Autodesk Fusion 360 part; units mm, degrees
note: some values were not read from the file. Set by a fixed rule: which face or edge a step refers to.
(part 3 of 5)
sketch "Sketch2 (10)" plane through (0, -26.65, 0) normal (0, -1, 0) x (1, 0, 0) in component "Front_R_Mounting_Plate"
  circle A0 centre (3, -97) radius 1.0625
  circle A1 centre (3, -71) radius 1.0625
  circle A2 centre (22, -71) radius 1.0625
  circle A3 centre (3, -29) radius 1.0625
  circle A4 centre (3, -3) radius 1.0625
  circle A5 centre (22, -29) radius 1.0625
  circle A6 centre (90, -16) radius 1.0625
  circle A7 centre (114, -16) radius 1.0625
  circle A8 centre (90, -30.28) radius 1.0625
  circle A9 centre (114, -30.28) radius 1.0625
  circle A10 centre (114, -69.72) radius 1.0625
  circle A11 centre (90, -84) radius 1.0625
  circle A12 centre (90, -69.72) radius 1.0625
  circle A13 centre (114, -84) radius 1.0625
  line L0 (92.5, -27.97) -> (92.5, -18.97)
  line L1 (92.5, -18.97) -> (112.5, -18.97)
  line L2 (112.5, -18.97) -> (112.5, -27.97)
  line L3 (112.5, -27.97) -> (92.5, -27.97)
  circle A14 centre (11.5, -70.07) radius 1
  circle A15 centre (11.5, -4.1) radius 1
  circle A16 centre (11.5, -29.93) radius 1
  line L4 (92.5, -81.36) -> (92.5, -72.36)
  line L5 (92.5, -72.36) -> (112.5, -72.36)
  line L6 (112.5, -72.36) -> (112.5, -81.36)
  line L7 (112.5, -81.36) -> (92.5, -81.36)
  circle A17 centre (89.585, -23.47) radius 1
  circle A18 centre (115.415, -76.86) radius 1
  line L8 (16, -72.97) -> (16, -93)
  line L9 (16, -93) -> (7, -93)
  line L10 (7, -93) -> (7, -72.97)
  line L11 (7, -72.97) -> (16, -72.97)
  line L12 (16, -7) -> (16, -27.03)
  line L13 (16, -27.03) -> (7, -27.03)
  line L14 (7, -27.03) -> (7, -7)
  line L15 (7, -7) -> (16, -7)
  circle A19 centre (11.5, -95.9) radius 1
  circle A20 centre (89.585, -76.86) radius 1
  circle A21 centre (115.415, -23.47) radius 1
  line L16 (127.5, -73.5) -> (124.5, -73.5)
  line L17 (124.5, -73.5) -> (124.5, -68.5)
  line L18 (124.5, -68.5) -> (127.5, -68.5)
  line L19 (127.5, -68.5) -> (127.5, -73.5)
  line L20 (183.5, -73.5) -> (180.5, -73.5)
  line L21 (180.5, -73.5) -> (180.5, -68.5)
  line L22 (180.5, -68.5) -> (183.5, -68.5)
  line L23 (183.5, -68.5) -> (183.5, -73.5)
  line L24 (127.5, -31.5) -> (124.5, -31.5)
  line L25 (124.5, -31.5) -> (124.5, -26.5)
  line L26 (124.5, -26.5) -> (127.5, -26.5)
  line L27 (127.5, -26.5) -> (127.5, -31.5)
  line L28 (183.5, -31.5) -> (180.5, -31.5)
  line L29 (180.5, -31.5) -> (180.5, -26.5)
  line L30 (180.5, -26.5) -> (183.5, -26.5)
  line L31 (183.5, -26.5) -> (183.5, -31.5)
  arc A22 (157, -3) -> (154, 0) centre (154, -3) ccw
  line L32 (154, 0) -> (3, 0)
  arc A23 (3, 0) -> (0, -3) centre (3, -3) ccw
  line L33 (0, -3) -> (0, -97)
  arc A24 (0, -97) -> (3, -100) centre (3, -97) ccw
  line L34 (3, -100) -> (154, -100)
  arc A25 (154, -100) -> (157, -97) centre (154, -97) ccw
  line L35 (157, -97) -> (157, -94)
  arc A26 (160, -91) -> (157, -94) centre (160, -94) ccw
  line L36 (160, -91) -> (181.27, -91)
  arc A27 (181.27, -91) -> (184.27, -88) centre (181.27, -88) ccw
  line L37 (184.27, -88) -> (184.27, -12)
  arc A28 (184.27, -12) -> (181.27, -9) centre (181.27, -12) ccw
  line L38 (181.27, -9) -> (160, -9)
  arc A29 (157, -6) -> (160, -9) centre (160, -6) ccw
  line L39 (157, -6) -> (157, -3)
  line L40 (36.83, -3.81) -> (36.83, -13.97)
  line L41 (36.83, -13.97) -> (19.05, -13.97)
  line L42 (19.05, -13.97) -> (19.05, -3.81)
  line L43 (19.05, -3.81) -> (36.83, -3.81)
  line L44 (36.83, -96.52) -> (19.05, -96.52)
  line L45 (19.05, -96.52) -> (19.05, -86.36)
  line L46 (19.05, -86.36) -> (36.83, -86.36)
  line L47 (36.83, -86.36) -> (36.83, -96.52)
  line L48 (114.3, -3.81) -> (130.81, -3.81)
  line L49 (130.81, -3.81) -> (130.81, -13.97)
  line L50 (130.81, -13.97) -> (114.3, -13.97)
  line L51 (114.3, -13.97) -> (114.3, -3.81)
  line L52 (114.3, -96.52) -> (114.3, -86.36)
  line L53 (114.3, -86.36) -> (130.81, -86.36)
  line L54 (130.81, -86.36) -> (130.81, -96.52)
  line L55 (130.81, -96.52) -> (114.3, -96.52)
  line L56 (25, -13.97) -> (25, -31.97)
  line L57 (25, -31.97) -> (0, -31.97)
  line L58 (0, -31.97) -> (0, -3)
  line L59 (19.05, -3.81) -> (19.05, 0)
  line L60 (19.05, 0) -> (3, 0)
  arc A30 (3, 0) -> (0, -3) centre (3, -3) ccw
  line L61 (19.05, -3.81) -> (19.05, -13.97)
  line L62 (19.05, -13.97) -> (25, -13.97)
  line L63 (7, -27.03) -> (7, -15.03) construction
  line L64 (7, -15.03) -> (16, -15.03)
  dimension "d323" = 25
  dimension "d324" = 18
  dimension "d325" = 3
  dimension "d326" = 12
  constraint coincident L41 L56.start
  constraint perpendicular L41 L56
  constraint coincident L33 L57.end
  constraint perpendicular L33 L57
  constraint coincident A23.end L33.start
  constraint coincident L42.end L43.start
  constraint coincident L32 L59.end
  constraint perpendicular L32 L59
  constraint coincident L32.end A23.start
  constraint coincident L41.end L42.start
  constraint coincident L13.end L14.start
  constraint perpendicular L13 L63
  constraint coincident L12 L64.end
  constraint perpendicular L12 L64
  measures "d323" distance of L56.end L57.end
  measures "d324" distance of L56.start L56.end
  measures "d325" radius of A30
  measures "d326" distance of L13.end L63.end
extrude "Extrude1''''''''''" add sketch "Sketch2 (10)" along normal blind 5.45 separate body contours A3 | A4 | A5 | L12 L14 L15 L64 | L32 A23 L33 L41 L42 L56 L57 L58 L59 L60 A30 L61 L62 makes body 15 in component "Front_R_Mounting_Plate"
sketch "Sketch3 (6)" plane through (0, -32.1, 0) normal (0, -1, 0) x (1, 0, 0) in component "Front_R_Mounting_Plate"
  line L0 (7, -27.03) -> (7, -15.03)
  line L1 (7, -15.03) -> (16, -15.03)
  line L2 (16, -15.03) -> (16, -27.03)
  line L3 (16, -27.03) -> (7, -27.03)
  line L4 (19.05, -13.97) -> (19.05, 0)
  line L5 (19.05, 0) -> (3, 0)
  arc A0 (3, 0) -> (0, -3) centre (3, -3) ccw
  line L6 (0, -3) -> (0, -31.97)
  line L7 (0, -31.97) -> (25, -31.97)
  line L8 (25, -31.97) -> (25, -13.97)
  line L9 (25, -13.97) -> (19.05, -13.97)
  line L10 (11.5, -27.03) -> (11.5, -23.23) construction
  circle A1 centre (11.5, -23.23) radius 8.2
  circle A2 centre (11.5, -23.23) radius 10.2
  circle A3 centre (11.5, -4.1) radius 1
  circle A4 centre (11.5, -29.93) radius 1
  dimension "d329" = 3.8
  dimension "d330" = 16.4
  dimension "d331" = 2
  constraint midpoint L3 L10.start
  constraint perpendicular L3 L10
  constraint coincident L10.end A1.centre
  measures "d329" distance of L10.start L10.end
  measures "d330" diameter of A1
extrude "Extrude2''''''''" cut sketch "Sketch3 (6)" against normal blind 2 contours L7 A2 picked at (9.2691, -14.4428) bodies 15 in component "Front_R_Mounting_Plate"
sketch "Sketch4 (7)" plane through (0, -26.65, 0) normal (0, -1, 0) x (1, 0, 0) in component "Front_R_Mounting_Plate"
  circle A0 centre (3, -97) radius 1.0625
  circle A1 centre (3, -71) radius 1.0625
  circle A2 centre (22, -71) radius 1.0625
  circle A3 centre (3, -29) radius 1.0625
  circle A4 centre (3, -3) radius 1.0625
  circle A5 centre (22, -29) radius 1.0625
  circle A6 centre (90, -16) radius 1.0625
  circle A7 centre (114, -16) radius 1.0625
  circle A8 centre (90, -30.28) radius 1.0625
  circle A9 centre (114, -30.28) radius 1.0625
  circle A10 centre (114, -69.72) radius 1.0625
  circle A11 centre (90, -84) radius 1.0625
  circle A12 centre (90, -69.72) radius 1.0625
  circle A13 centre (114, -84) radius 1.0625
  line L0 (92.5, -27.97) -> (92.5, -18.97)
  line L1 (92.5, -18.97) -> (112.5, -18.97)
  line L2 (112.5, -18.97) -> (112.5, -27.97)
  line L3 (112.5, -27.97) -> (92.5, -27.97)
  circle A14 centre (11.5, -70.07) radius 1
  circle A15 centre (11.5, -4.1) radius 1
  circle A16 centre (11.5, -29.93) radius 1
  line L4 (92.5, -81.36) -> (92.5, -72.36)
  line L5 (92.5, -72.36) -> (112.5, -72.36)
  line L6 (112.5, -72.36) -> (112.5, -81.36)
  line L7 (112.5, -81.36) -> (92.5, -81.36)
  circle A17 centre (89.585, -23.47) radius 1
  circle A18 centre (115.415, -76.86) radius 1
  line L8 (16, -72.97) -> (16, -93)
  line L9 (16, -93) -> (7, -93)
  line L10 (7, -93) -> (7, -72.97)
  line L11 (7, -72.97) -> (16, -72.97)
  line L12 (16, -7) -> (16, -27.03)
  line L13 (16, -27.03) -> (7, -27.03)
  line L14 (7, -27.03) -> (7, -7)
  line L15 (7, -7) -> (16, -7)
  circle A19 centre (11.5, -95.9) radius 1
  circle A20 centre (89.585, -76.86) radius 1
  circle A21 centre (115.415, -23.47) radius 1
  line L16 (127.5, -73.5) -> (124.5, -73.5)
  line L17 (124.5, -73.5) -> (124.5, -68.5)
  line L18 (124.5, -68.5) -> (127.5, -68.5)
  line L19 (127.5, -68.5) -> (127.5, -73.5)
  line L20 (183.5, -73.5) -> (180.5, -73.5)
  line L21 (180.5, -73.5) -> (180.5, -68.5)
  line L22 (180.5, -68.5) -> (183.5, -68.5)
  line L23 (183.5, -68.5) -> (183.5, -73.5)
  line L24 (127.5, -31.5) -> (124.5, -31.5)
  line L25 (124.5, -31.5) -> (124.5, -26.5)
  line L26 (124.5, -26.5) -> (127.5, -26.5)
  line L27 (127.5, -26.5) -> (127.5, -31.5)
  line L28 (183.5, -31.5) -> (180.5, -31.5)
  line L29 (180.5, -31.5) -> (180.5, -26.5)
  line L30 (180.5, -26.5) -> (183.5, -26.5)
  line L31 (183.5, -26.5) -> (183.5, -31.5)
  arc A22 (157, -3) -> (154, 0) centre (154, -3) ccw
  line L32 (154, 0) -> (3, 0)
  arc A23 (3, 0) -> (0, -3) centre (3, -3) ccw
  line L33 (0, -3) -> (0, -97)
  arc A24 (0, -97) -> (3, -100) centre (3, -97) ccw
  line L34 (3, -100) -> (154, -100)
  arc A25 (154, -100) -> (157, -97) centre (154, -97) ccw
  line L35 (157, -97) -> (157, -94)
  arc A26 (160, -91) -> (157, -94) centre (160, -94) ccw
  line L36 (160, -91) -> (181.27, -91)
  arc A27 (181.27, -91) -> (184.27, -88) centre (181.27, -88) ccw
  line L37 (184.27, -88) -> (184.27, -12)
  arc A28 (184.27, -12) -> (181.27, -9) centre (181.27, -12) ccw
  line L38 (181.27, -9) -> (160, -9)
  arc A29 (157, -6) -> (160, -9) centre (160, -6) ccw
  line L39 (157, -6) -> (157, -3)
  line L40 (36.83, -3.81) -> (36.83, -13.97)
  line L41 (36.83, -13.97) -> (19.05, -13.97)
  line L42 (19.05, -13.97) -> (19.05, -3.81)
  line L43 (19.05, -3.81) -> (36.83, -3.81)
  line L44 (36.83, -96.52) -> (19.05, -96.52)
  line L45 (19.05, -96.52) -> (19.05, -86.36)
  line L46 (19.05, -86.36) -> (36.83, -86.36)
  line L47 (36.83, -86.36) -> (36.83, -96.52)
  line L48 (114.3, -3.81) -> (130.81, -3.81)
  line L49 (130.81, -3.81) -> (130.81, -13.97)
  line L50 (130.81, -13.97) -> (114.3, -13.97)
  line L51 (114.3, -13.97) -> (114.3, -3.81)
  line L52 (114.3, -96.52) -> (114.3, -86.36)
  line L53 (114.3, -86.36) -> (130.81, -86.36)
  line L54 (130.81, -86.36) -> (130.81, -96.52)
  line L55 (130.81, -96.52) -> (114.3, -96.52)
  circle A30 centre (3, -29) radius 1.0625
  circle A31 centre (22, -29) radius 1.0625
  circle A32 centre (3, -3) radius 1.0625
  circle A33 centre (3, -3) radius 1.0625
  circle A34 centre (3, -3) radius 1.0625
  circle A35 centre (22, -29) radius 1.0625
  circle A36 centre (3, -29) radius 1.0625
  circle A37 centre (3, -3) radius 1.0625
  circle A38 centre (3, -3) radius 1.0625
  circle A39 centre (3, -3) radius 0.95
  circle A40 centre (3, -29) radius 0.95
  circle A41 centre (22, -29) radius 0.95
  dimension "d334" = 1.9
  dimension "d335" = 1.9
  dimension "d336" = 1.9
  constraint concentric A36 A40
  constraint concentric A35 A41
  measures "d334" diameter of A39
  measures "d335" diameter of A40
  measures "d336" diameter of A41
extrude "Extrude3''''''" add sketch "Sketch4 (7)" against normal blind 1 contours A39 | A40 | A41 bodies 15 in component "Front_R_Mounting_Plate"
sketch "Sketch6 (4)" plane through (0, -26.65, 0) normal (0, 1, 0) x (-1, 0, 0) in component "Front_R_Mounting_Plate"
  circle A0 centre (-22, -29) radius 0.95
  circle A1 centre (-3, -3) radius 0.95
  circle A2 centre (-3, -29) radius 0.95
  line L0 (-7, -15.03) -> (-7, -27.03)
  line L1 (-7, -27.03) -> (-16, -27.03)
  line L2 (-16, -27.03) -> (-16, -15.03)
  line L3 (-16, -15.03) -> (-7, -15.03)
  line L4 (-19.05, 0) -> (-19.05, -13.97)
  line L5 (-19.05, -13.97) -> (-25, -13.97)
  line L6 (-25, -13.97) -> (-25, -31.97)
  line L7 (-25, -31.97) -> (0, -31.97)
  line L8 (0, -31.97) -> (0, -3)
  arc A3 (0, -3) -> (-3, 0) centre (-3, -3) ccw
  line L9 (-3, 0) -> (-19.05, 0)
  line L10 (-17.55, 0) -> (-5.45, 0)
  line L11 (-5.45, 0) -> (-5.45, -31.97)
  line L12 (-17.55, -31.97) -> (-17.55, 0)
  line L13 (-17.55, 0) -> (-8.3527, -31.97) construction
  line L14 (-5.45, 0) -> (-14.6473, -31.97) construction
  line L15 (-5.45, -31.97) -> (-17.55, -31.97)
  circle A4 centre (-11.5, -4.1) radius 1
  circle A5 centre (-11.5, -29.93) radius 1
  point P0 (-11.5, -21.03)
  dimension "d340" = 7.45
  dimension "d341" = 5.45
  constraint horizontal L10
  constraint perpendicular L10 L11
  constraint parallel L11 L12
  constraint coincident L13 P0
  constraint coincident L14 P0
  constraint coincident L7 L14.end
  constraint coincident L7 L13.end
  constraint coincident L7 L11.end
  constraint coincident L7 L12.start
  measures "d340" distance of L6 L12
  measures "d341" distance of L8 L11
extrude "Extrude4''''''" cut sketch "Sketch6 (4)" against normal blind 1.5 contours L7 L9 L10 L11 L12 L15 | A4 | A5 bodies 15 in component "Front_R_Mounting_Plate"
extrude "Extrude18''" add 4 faces at (92.6744, -34.28, -80.7632) (100.2032, -34.28, -80.4856) (99.9256, -34.28, -72.9568) (92.3968, -34.28, -73.2344) along direction (0, 1, 0) blind 1.8 on bodies 12 bodies 12 in component "Back_Wheel_L"
extrude "Extrude19''" add 8 faces at (91.0152, -35.28, -77.0342) (94.3333, -35.28, -74.9002) (96.4742, -35.28, -71.5752) (98.2598, -35.28, -74.8933) (101.59, -35.28, -76.86) (98.2598, -35.28, -78.8267) (96.4742, -35.28, -82.1448) (94.3333, -35.28, -78.8198) along direction (0, 1, 0) blind 1.8 on bodies 12 bodies 12 in component "Back_Wheel_L"
extrude "Extrude20'" add 4 faces at (92.6744, -34.28, -80.7632) (100.2032, -34.28, -80.4856) (99.9256, -34.28, -72.9568) (92.3968, -34.28, -73.2344) along direction (0, 1, 0) blind 1.8 on bodies 13 bodies 13 in component "Back_Wheel_R"
extrude "Extrude21" add 8 faces at (91.0152, -35.28, -77.0342) (94.3333, -35.28, -74.9002) (96.4742, -35.28, -71.5752) (98.2598, -35.28, -74.8933) (101.59, -35.28, -76.86) (98.2598, -35.28, -78.8267) (96.4742, -35.28, -82.1448) (94.3333, -35.28, -78.8198) along direction (0, 1, 0) blind 1.8 on bodies 13 bodies 13 in component "Back_Wheel_R"
sketch "Sketch50" plane through (0, -33.48, 0) normal (0, 1, 0) x (-1, 0, 0)
  circle A0 centre (-96.3, -76.86) radius 2.25
  arc A1 (-97.86, -80.42) -> (-99.86, -78.42) centre (-99.86, -80.42) ccw
  line L0 (-97.86, -80.42) -> (-97.86, -85.4698)
  arc A2 (-97.86, -85.4698) -> (-94.74, -85.4698) centre (-96.3, -76.86) ccw
  line L1 (-94.74, -85.4698) -> (-94.74, -80.42)
  arc A3 (-92.74, -78.42) -> (-94.74, -80.42) centre (-92.74, -80.42) ccw
  line L2 (-92.74, -78.42) -> (-87.6902, -78.42)
  arc A4 (-87.6902, -78.42) -> (-87.6902, -75.3) centre (-96.3, -76.86) ccw
  line L3 (-87.6902, -75.3) -> (-92.74, -75.3)
  arc A5 (-94.74, -73.3) -> (-92.74, -75.3) centre (-92.74, -73.3) ccw
  line L4 (-94.74, -73.3) -> (-94.74, -68.2502)
  arc A6 (-94.74, -68.2502) -> (-97.86, -68.2502) centre (-96.3, -76.86) ccw
  line L5 (-97.86, -68.2502) -> (-97.86, -73.3)
  arc A7 (-99.86, -75.3) -> (-97.86, -73.3) centre (-99.86, -73.3) ccw
  line L6 (-99.86, -75.3) -> (-104.9098, -75.3)
  arc A8 (-104.9098, -75.3) -> (-104.9098, -78.42) centre (-96.3, -76.86) ccw
  line L7 (-104.9098, -78.42) -> (-99.86, -78.42)
  line L8 (-96.8, -80.3599) -> (-96.8, -85)
  line L9 (-95.8, -80.3601) -> (-95.8, -85)
  arc A9 (-96.8, -85) -> (-95.8, -85) centre (-96.3, -85) ccw
  arc A10 (-95.8, -80.3601) -> (-96.8, -80.3599) centre (-96.3, -80.36) ccw
  line L10 (-105.05, -76.86) -> (-87.55, -76.86) construction
  line L11 (-95.8, -73.3599) -> (-95.8, -68.72)
  arc A11 (-95.8, -68.72) -> (-96.8, -68.72) centre (-96.3, -68.72) ccw
  line L12 (-96.8, -73.3601) -> (-96.8, -68.72)
  arc A12 (-96.8, -73.3601) -> (-95.8, -73.3599) centre (-96.3, -73.36) ccw
  line L13 (-88.16, -77.36) -> (-92.8, -77.36)
  line L14 (-88.16, -76.36) -> (-92.8, -76.36)
  line L15 (-96.3, -79.11) -> (-96.3, -85.61) construction
  arc A13 (-92.8, -76.36) -> (-92.8, -77.36) centre (-92.8, -76.86) ccw
  arc A14 (-88.16, -77.36) -> (-88.16, -76.36) centre (-88.16, -76.86) ccw
  line L16 (-104.44, -77.36) -> (-99.8, -77.36)
  arc A15 (-99.8, -77.36) -> (-99.8, -76.36) centre (-99.8, -76.86) ccw
  line L17 (-104.44, -76.36) -> (-99.8, -76.36)
  arc A16 (-104.44, -76.36) -> (-104.44, -77.36) centre (-104.44, -76.86) ccw
  dimension "d352" = 1
  dimension "d353" = 1
  dimension "d354" = 3.5
  dimension "d355" = 1.06
  dimension "d356" = 4.6399
  dimension "d357" = 1
  dimension "d358" = 8.14
  dimension "d359" = 3.5
  dimension "d360" = 1
  dimension "d361" = 8.14
  constraint tangent L8 A9
  constraint tangent L9 A9
  constraint midpoint A8 L10.start
  constraint midpoint A4 L10.end
  constraint symmetric L9.start L10 L11.start
  constraint symmetric L8.start L10 L12.start
  constraint symmetric L8.end L10 A11.end
  constraint symmetric L9.end L10 L11.end
  constraint symmetric A9 L10 A11
  constraint symmetric A10 L10 A12
  constraint coincident L10 A13.centre
  constraint coincident L10 A14.centre
  constraint tangent L13 A13
  constraint tangent L14 A13
  constraint midpoint A2 L15.end
  constraint coincident A0 L15.start
  constraint symmetric L13.start L15 L16.start
  constraint symmetric L14.start L15 L17.start
  constraint symmetric L13.end L15 L16.end
  constraint symmetric L14.end L15 A15.end
  constraint symmetric L15 A13 A15
  constraint symmetric L15 A14 A16
  measures "d352" diameter of A10
  measures "d353" diameter of A9
  measures "d354" distance of A0.centre A10.centre
  measures "d355" distance of L0 L8
  measures "d356" distance of L9.start L9.end
  measures "d357" diameter of A13
  measures "d358" vertical distance of A0.centre A9.centre
  measures "d359" distance of A0.centre A13.centre
  measures "d360" diameter of A14
  measures "d361" distance of A0.centre A14.centre
extrude "Extrude20''" cut sketch "Sketch50" against normal blind 2.8 contours L8 L9 A9 A10 | L11 A11 L12 A12 | L13 L14 A13 A14 | L16 A15 L17 A16 bodies 12 in component "Back_Wheel_L"
sketch "Sketch18 (2)" plane through (0, -33.48, 0) normal (0, 1, 0) x (-1, 0, 0) in component "Back_Wheel_R"
  line L0 (-94.74, -73.3) -> (-94.74, -68.2502)
  arc A0 (-94.74, -68.2502) -> (-97.86, -68.2502) centre (-96.3, -76.86) ccw
  line L1 (-97.86, -68.2502) -> (-97.86, -73.3)
  arc A1 (-99.86, -75.3) -> (-97.86, -73.3) centre (-99.86, -73.3) ccw
  line L2 (-99.86, -75.3) -> (-104.9098, -75.3)
  arc A2 (-104.9098, -75.3) -> (-104.9098, -78.42) centre (-96.3, -76.86) ccw
  line L3 (-104.9098, -78.42) -> (-99.86, -78.42)
  arc A3 (-97.86, -80.42) -> (-99.86, -78.42) centre (-99.86, -80.42) ccw
  line L4 (-97.86, -80.42) -> (-97.86, -85.4698)
  arc A4 (-97.86, -85.4698) -> (-94.74, -85.4698) centre (-96.3, -76.86) ccw
  line L5 (-94.74, -85.4698) -> (-94.74, -80.42)
  arc A5 (-92.74, -78.42) -> (-94.74, -80.42) centre (-92.74, -80.42) ccw
  line L6 (-92.74, -78.42) -> (-87.6902, -78.42)
  arc A6 (-87.6902, -78.42) -> (-87.6902, -75.3) centre (-96.3, -76.86) ccw
  line L7 (-87.6902, -75.3) -> (-92.74, -75.3)
  arc A7 (-94.74, -73.3) -> (-92.74, -75.3) centre (-92.74, -73.3) ccw
  circle A8 centre (-96.3, -76.86) radius 2.25
  line L8 (-96.3, -76.86) -> (-96.3, -73.36) construction
  line L9 (-96.3, -76.86) -> (-92.8, -76.86)
  line L10 (-92.8, -76.86) -> (-92.8, -77.36) construction
  line L11 (-92.8, -76.86) -> (-92.8, -76.36) construction
  line L12 (-96.3, -73.36) -> (-96.8, -73.36) construction
  line L13 (-96.3, -73.36) -> (-95.8, -73.36) construction
  line L14 (-92.8, -77.36) -> (-88.16, -77.36)
  line L15 (-92.8, -76.36) -> (-88.16, -76.36)
  arc A9 (-88.16, -77.36) -> (-88.16, -76.36) centre (-88.16, -76.86) ccw
  arc A10 (-92.8, -76.36) -> (-92.8, -77.36) centre (-92.8, -76.86) ccw
  line L16 (-95.8, -73.36) -> (-95.8, -68.72)
  line L17 (-96.8, -73.36) -> (-96.8, -68.72)
  arc A11 (-96.8, -73.36) -> (-95.8, -73.36) centre (-96.3, -73.36) ccw
  arc A12 (-95.8, -68.72) -> (-96.8, -68.72) centre (-96.3, -68.72) ccw
  line L18 (-96.3, -76.86) -> (-100, -76.86) construction
  line L19 (-96.3, -76.86) -> (-96.3, -80) construction
  line L20 (-99.8, -77.36) -> (-104.44, -77.36)
  arc A13 (-104.44, -76.36) -> (-104.44, -77.36) centre (-104.44, -76.86) ccw
  line L21 (-99.8, -76.36) -> (-104.44, -76.36)
  arc A14 (-99.8, -77.36) -> (-99.8, -76.36) centre (-99.8, -76.86) ccw
  line L22 (-96.8, -80.36) -> (-96.8, -85)
  arc A15 (-95.8, -80.36) -> (-96.8, -80.36) centre (-96.3, -80.36) ccw
  line L23 (-95.8, -80.36) -> (-95.8, -85)
  arc A16 (-96.8, -85) -> (-95.8, -85) centre (-96.3, -85) ccw
  dimension "d364" = 3.5
  dimension "d365" = 3.5
  dimension "d366" = 1
  dimension "d367" = 1
  dimension "d368" = 1
  dimension "d369" = 1
  dimension "d370" = 8.14
  dimension "d371" = 8.14
  constraint coincident A0.centre A2.centre
  constraint vertical L8
  constraint perpendicular L8 L9
  constraint coincident L9.end L10.start
  constraint coincident L8.end L12.start
  constraint perpendicular L9 L10
  constraint perpendicular L9 L11
  constraint perpendicular L8 L12
  constraint perpendicular L8 L13
  constraint tangent L14 A9
  constraint perpendicular L10 L14
  constraint tangent L15 A9
  constraint tangent L16 A12
  constraint perpendicular L13 L16
  constraint tangent L17 A12
  constraint perpendicular L8 L18
  constraint perpendicular L18 L19
  constraint symmetric L10.end L19 L20.start
  constraint symmetric L11.end L19 L21.start
  constraint symmetric L14.end L19 L20.end
  constraint symmetric L15.end L19 A13.start
  constraint symmetric A9 L19 A13
  constraint symmetric A10 L19 A14
  constraint symmetric L12.end L18 L22.start
  constraint symmetric L13.end L18 A15.start
  constraint symmetric L16.end L18 L23.end
  constraint symmetric L17.end L18 L22.end
  constraint symmetric A11 L18 A15
  constraint symmetric A12 L18 A16
  measures "d364" distance of A0.centre L8.end
  measures "d365" distance of A0.centre L9.end
  measures "d366" diameter of A10
  measures "d367" diameter of A11
  measures "d368" diameter of A9
  measures "d369" diameter of A12
  measures "d370" distance of A0.centre A9.centre
  measures "d371" distance of A0.centre A12.centre
extrude "Extrude22" cut sketch "Sketch18 (2)" against normal blind 2.8 contours L14 L15 A9 A10 | L16 L17 A11 A12 | L20 A13 L21 A14 | L22 A15 L23 A16 bodies 13 in component "Back_Wheel_R"
extrude "Extrude21'" cut 4 faces at (100.2032, -32.48, -80.4856) (92.6744, -32.48, -80.7632) (99.9256, -32.48, -72.9568) (92.3968, -32.48, -73.2344) along direction (0, -1, 0) blind 0.75 on bodies 12 bodies 12 in component "Back_Wheel_L"
extrude "Extrude22'" cut 1 faces at (95.0933, -33.48, -83.6299) along direction (0, -1, 0) blind 0.75 on bodies 12 bodies 12 in component "Back_Wheel_L"
extrude "Extrude23" cut 1 faces at (89.5301, -33.48, -75.6533) along direction (0, -1, 0) blind 0.75 on bodies 13 bodies 13 in component "Back_Wheel_R"
extrude "Extrude24" cut 4 faces at (99.9256, -32.48, -72.9568) (92.3968, -32.48, -73.2344) (100.2032, -32.48, -80.4856) (92.6744, -32.48, -80.7632) along direction (0, -1, 0) blind 0.75 on bodies 13 bodies 13 in component "Back_Wheel_R"
extrude "Extrude23'" add 1 faces at (94.9011, -36.28, -70.2649) along direction (0, -1, 0) blind 0.95 on bodies 12 bodies 12 in component "Back_Wheel_L"
extrude "Extrude25" add 1 faces at (97.6989, -36.28, -83.455) along direction (0, -1, 0) blind 0.95 on bodies 13 bodies 13 in component "Back_Wheel_R"
sketch "Sketch1 (9)" plane through (0, 1.57, 0) normal (0, 1, 0) x (-1, 0, 0) in component "LCD_Mount"
  line L0 (-36.83, -3.81) -> (-19.05, -3.81)
  line L1 (-19.05, -3.81) -> (-19.05, -13.97)
  line L2 (-19.05, -13.97) -> (-36.83, -13.97)
  line L3 (-36.83, -13.97) -> (-36.83, -3.81)
  circle A0 centre (-122.9106, -82.4992) radius 2.54
  circle A1 centre (-52.2224, -92.0496) radius 2.54
  line L4 (-114.3, -96.52) -> (-130.81, -96.52)
  line L5 (-130.81, -96.52) -> (-130.81, -86.36)
  line L6 (-130.81, -86.36) -> (-114.3, -86.36)
  line L7 (-114.3, -86.36) -> (-114.3, -96.52)
  line L8 (-36.83, -96.52) -> (-36.83, -86.36)
  line L9 (-36.83, -86.36) -> (-19.05, -86.36)
  line L10 (-19.05, -86.36) -> (-19.05, -96.52)
  line L11 (-19.05, -96.52) -> (-36.83, -96.52)
  circle A2 centre (-102.5398, -7.1374) radius 2.54
  circle A3 centre (-21.2344, -29.4894) radius 2.54
  circle A4 centre (-147.6502, -58.6486) radius 2.54
  line L12 (-114.3, -3.81) -> (-114.3, -13.97) construction
  line L13 (-114.3, -13.97) -> (-130.81, -13.97)
  line L14 (-130.81, -13.97) -> (-130.81, -3.81)
  line L15 (-130.81, -3.81) -> (-114.3, -3.81)
  line L16 (0, -100) -> (0, 0)
  line L17 (0, 0) -> (-160, 0)
  line L18 (-160, 0) -> (-160, -100)
  line L19 (-160, -100) -> (0, -100)
  line L20 (-119.0032, -3.81) -> (-98, -3.81)
  line L21 (-98, -3.81) -> (-98, -11.0959)
  line L22 (-98, -11.0959) -> (-114.3, -13.97)
  line L23 (-114.3, -13.97) -> (-119, -13.97)
  line L24 (-119, -13.97) -> (-119.0032, -3.81)
  circle A5 centre (-102.5398, -7.1374) radius 2.75
  dimension "d386" = 100
  dimension "d389" = 5.5
  constraint coincident L15 L20.start
  constraint parallel L15 L20
  constraint perpendicular L15 L21
  constraint coincident L12.end L13.start
  constraint coincident L13 L23.end
  constraint perpendicular L12 L23
  constraint concentric A2 A5
  measures "d386" angle of L21 L22
  measures "d389" diameter of A5
extrude "Extrude2'''''''''" add sketch "Sketch1 (9)" along normal blind 3 separate body contours L13 L15 L20 L21 L22 L23 L24 makes body 16 in component "LCD_Mount"
extrude "Extrude1'''''''''''" add sketch "Sketch1 (9)" along normal blind 3 separate body contours L13 L15 L20 L21 L22 L23 L24 | A5 makes body 17 in component "LCD_Mount"
sketch "Sketch4 (8)" plane through (0, 1.57, 0) normal (0, -1, 0) x (1, 0, 0) in component "LCD_Mount"
  circle A0 centre (102.5398, -7.1374) radius 2.54
  line L0 (114.3, -13.97) -> (119, -13.97)
  line L1 (119, -13.97) -> (119.0032, -3.81)
  line L2 (119.0032, -3.81) -> (98, -3.81)
  line L3 (98, -3.81) -> (98, -11.0959)
  line L4 (98, -11.0959) -> (114.3, -13.97)
  line L5 (119, -13.97) -> (114.32, -13.97)
  line L6 (114.32, -13.97) -> (114.32, -3.81)
  line L7 (114.32, -3.81) -> (119, -3.81)
  line L8 (119, -3.81) -> (119, -13.97)
  dimension "d392" = 4.68
  constraint horizontal L5
  constraint vertical L6
  constraint horizontal L7
  constraint vertical L8
  constraint coincident L2 L6.end
  constraint coincident L0.end L1.start
  measures "d392" distance of L0.end L5.end
extrude "Extrude3'''''''" add sketch "Sketch4 (8)" along normal blind 1.57 contours L0 L2 L5 L6 L7 L8 bodies 16 17 in component "LCD_Mount"
sketch "Sketch5 (5)" plane through (0, 4.57, 0) normal (0, 1, 0) x (-1, 0, 0) in component "LCD_Mount"
  circle A0 centre (-102.5398, -7.1374) radius 2.54
  line L0 (-119, -13.97) -> (-114.3, -13.97)
  line L1 (-114.3, -13.97) -> (-98, -11.0959)
  line L2 (-98, -11.0959) -> (-98, -3.81)
  line L3 (-98, -3.81) -> (-119.0032, -3.81)
  line L4 (-119.0032, -3.81) -> (-119, -13.97)
  line L5 (-119.0032, -3.81) -> (-114.3, -3.81)
  line L6 (-114.3, -3.81) -> (-114.3, -13.97)
  line L7 (-114.3, -13.97) -> (-119.0032, -13.97)
  line L8 (-119.0032, -13.97) -> (-119.0032, -3.81)
  constraint horizontal L5
  constraint vertical L6
  constraint horizontal L7
  constraint vertical L8
  constraint coincident L0.end L1.start
  constraint coincident L3.end L4.start
extrude "Extrude4'''''''" add sketch "Sketch5 (5)" along normal blind 50 contours L0 L3 L4 L5 L6 L7 bodies 16 in component "LCD_Mount"
sketch "Sketch6 (5)" plane through (0, 0, -13.97) normal (0, 0, -1) x (-1, 0, 0) in component "LCD_Mount"
  line L0 (-119, 1.57) -> (-119, 0)
  line L1 (-119, 0) -> (-114.32, 0)
  line L2 (-114.32, 0) -> (-114.32, 1.57)
  line L3 (-114.32, 1.57) -> (-114.3, 1.57)
  line L4 (-114.3, 1.57) -> (-114.3, 4.57)
  line L5 (-114.3, 4.57) -> (-114.3, 54.57)
  line L6 (-114.3, 54.57) -> (-119, 54.57)
  line L7 (-119, 54.57) -> (-119, 1.57)
  line L8 (-114.3, 54.57) -> (-105.4984, 42)
  line L9 (-105.4984, 42) -> (-119, 42)
  line L10 (-119, 42) -> (-119, 54.57)
  line L11 (-119, 54.57) -> (-114.3, 54.57)
  dimension "d397" = 35
  dimension "d398" = 13.5016
  constraint coincident L5.end L6.start
  constraint coincident L7 L9.end
  constraint perpendicular L7 L9
  constraint coincident L6.end L7.start
  measures "d397" angle of L5 L8
  measures "d398" distance of L8.end L9.end
extrude "Extrude5''''" add sketch "Sketch6 (5)" along normal blind 50 contours L5 L6 L7 L9 L10 L11 | L5 L8 L9 bodies 16 in component "LCD_Mount"
sketch "Sketch7 (3)" plane through (51.0569, -35.7505, 0) normal (-0.819152, 0.573576, 0) x (0, 0, 1) in component "LCD_Mount"
  line L0 (-13.97, 94.9158) -> (-13.97, 110.2609)
  line L1 (-13.97, 110.2609) -> (-63.97, 110.2609)
  line L2 (-63.97, 110.2609) -> (-63.97, 94.9158)
  line L3 (-63.97, 94.9158) -> (-13.97, 94.9158)
  line L4 (-14.97, 95.9158) -> (-14.97, 109.2609)
  line L5 (-14.97, 109.2609) -> (-62.97, 109.2609)
  line L6 (-62.97, 109.2609) -> (-62.97, 95.9158)
  line L7 (-62.97, 95.9158) -> (-62.97, 94.9158)
  line L8 (-14.97, 95.9158) -> (-14.97, 94.9158)
  circle A0 centre (-54.21, 102.5883) radius 1.3
  circle A1 centre (-23.73, 102.5883) radius 1.3
  line L9 (-38.97, 109.2609) -> (-38.97, 94.9158) construction
  line L10 (-62.97, 102.5883) -> (-14.97, 102.5883) construction
  line L11 (-51.71, 100.0883) -> (-56.71, 100.0883)
  line L12 (-56.71, 100.0883) -> (-56.71, 105.0883)
  line L13 (-56.71, 105.0883) -> (-51.71, 105.0883)
  line L14 (-51.71, 105.0883) -> (-51.71, 100.0883)
  line L15 (-51.71, 100.0883) -> (-56.71, 105.0883) construction
  line L16 (-56.71, 100.0883) -> (-51.71, 105.0883) construction
  line L17 (-21.23, 100.0883) -> (-26.23, 100.0883)
  line L18 (-26.23, 100.0883) -> (-26.23, 105.0883)
  line L19 (-26.23, 105.0883) -> (-21.23, 105.0883)
  line L20 (-21.23, 105.0883) -> (-21.23, 100.0883)
  line L21 (-21.23, 100.0883) -> (-26.23, 105.0883) construction
  line L22 (-26.23, 100.0883) -> (-21.23, 105.0883) construction
  point P0 (-54.21, 102.5883)
  point P1 (-23.73, 102.5883)
  dimension "d402" = 13.3451
  dimension "d403" = 48
  dimension "d404" = 13.3451
  dimension "d405" = 1
  dimension "d406" = 1
  dimension "d407" = 2.6
  dimension "d408" = 2.6
  dimension "d409" = 30.48
  dimension "d410" = 5
  dimension "d411" = 5
  dimension "d412" = 5
  dimension "d413" = 5
  constraint coincident L3 L7.end
  constraint perpendicular L3 L7
  constraint coincident L3 L8.end
  constraint perpendicular L3 L8
  constraint parallel L0 L4
  constraint parallel L1 L5
  constraint parallel L2 L6
  constraint horizontal P0 P1
  constraint midpoint L5 L9.start
  constraint midpoint L3 L9.end
  constraint symmetric P0 P1 L9
  constraint midpoint L6 L10.start
  constraint midpoint L4 L10.end
  constraint coincident P0 L10
  constraint horizontal L11
  constraint perpendicular L11 L12
  constraint parallel L11 L13
  constraint parallel L12 L14
  constraint coincident L15 P0
  constraint coincident L16 P0
  constraint coincident P0 A0.centre
  constraint horizontal L17
  constraint perpendicular L17 L18
  constraint parallel L17 L19
  constraint parallel L18 L20
  constraint coincident L21 P1
  constraint coincident L22 P1
  constraint coincident P1 A1.centre
  measures "d402" distance of L6.end L5.end
  measures "d403" distance of L4.end L5.end
  measures "d404" distance of L4.start L4.end
  measures "d405" distance of L1 L5
  measures "d406" distance of L2 L6
  measures "d407" diameter of A0
  measures "d408" diameter of A1
  measures "d409" horizontal distance of P0 P1
  measures "d410" distance of L12.end L13.end
  measures "d411" distance of L11.end L12.end
  measures "d412" distance of L18.end L19.end
  measures "d413" distance of L17.end L18.end
extrude "Extrude6''''" cut sketch "Sketch7 (3)" against normal blind 1.5 contours L3 L4 L5 L6 L7 L8 bodies 16 in component "LCD_Mount"
extrude "Extrude7'" cut sketch "Sketch7 (3)" against normal blind 23 contours A0 | A1 bodies 16 in component "LCD_Mount"
chamfer "Chamfer1" distance 4 angle 45 3 edges at (119, 42, -18.201) (119, 42, -38.97) (119, 42, -59.739) on bodies 16 in component "LCD_Mount"
extrude "Extrude8'" cut 1 faces at (110.2404, 47.0288, -26.23) along direction (0, 0, 1) blind 0.75 on bodies 16 bodies 16 in component "LCD_Mount"
extrude "Extrude9'" cut 1 faces at (111.1963, 48.3941, -51.71) along direction (0, 0, -1) blind 0.75 on bodies 16 bodies 16 in component "LCD_Mount"
sketch "Sketch20" plane through (0, 0, -100) normal (0, 0, -1) x (-1, 0, 0) in component "Chassis"
  circle A0 centre (-122.5668, -10.65) radius 1.25
  circle A1 centre (-122.5668, -5.65) radius 1.25
  line L0 (-154, 0) -> (-154, -26.65)
  line L1 (-154, -26.65) -> (-3, -26.65)
  line L2 (-3, -26.65) -> (-3, 0)
  line L3 (-3, 0) -> (-154, 0)
  line L4 (-3, -26.65) -> (-28, -26.65)
  line L5 (-28, -26.65) -> (-28, 0)
  line L6 (-28, 0) -> (-3, 0)
  line L7 (-3, 0) -> (-3, -26.65)
  dimension "d423" = 25
  dimension "d424" = 26.65
  constraint horizontal L4
  constraint vertical L5
  constraint horizontal L6
  constraint vertical L7
  constraint coincident L1.end L2.start
  measures "d423" distance of L1.end L4.end
  measures "d424" distance of L1.end L2.end
extrude "Extrude21''" add sketch "Sketch20" along normal blind 3 contours L1 L2 L3 L4 L5 L6 L7 bodies 4 in component "Chassis"
chamfer "Chamfer1'" distance 3 angle 45 1 edges at (28, -13.325, -103) on bodies 4 in component "Chassis"
sketch "Sketch21" plane through (0, 0, 0) normal (0, 0, 1) x (1, 0, 0) in component "Chassis"
  line L0 (154, -26.65) -> (154, 0)
  line L1 (154, 0) -> (3, 0)
  line L2 (3, 0) -> (3, -26.65)
  line L3 (3, -26.65) -> (154, -26.65)
  line L4 (3, -26.65) -> (28, -26.65)
  line L5 (28, -26.65) -> (28, 0)
  line L6 (28, 0) -> (3, 0)
  line L7 (3, 0) -> (3, -26.65)
  dimension "d429" = 25
  constraint horizontal L4
  constraint vertical L5
  constraint horizontal L6
  constraint vertical L7
  constraint coincident L2.end L3.start
  measures "d429" distance of L2.end L4.end
extrude "Extrude22''" add sketch "Sketch21" along normal blind 3 contours L1 L2 L3 L4 L5 L6 L7 bodies 4 in component "Chassis"
chamfer "Chamfer2" distance 3 angle 45 1 edges at (3, -13.325, 3) on bodies 4 in component "Chassis"
chamfer "Chamfer3" distance 3 angle 45 1 edges at (28, -13.325, 3) on bodies 4 in component "Chassis"
chamfer "Chamfer4" distance 3 angle 45 1 edges at (3, -13.325, -103) on bodies 4 in component "Chassis"
sketch "Sketch22" plane through (0, 0, 0) normal (0, 1, 0) x (-1, 0, 0) in component "Chassis"
  line L0 (-6, -103) -> (-3, -100)
  arc A0 (-3, -100) -> (0, -97) centre (-3, -97) ccw
  line L1 (0, -97) -> (0, -94)
  line L2 (0, -94) -> (-3, -94)
  arc A1 (-6, -97) -> (-3, -94) centre (-6, -94) ccw
  line L3 (-6, -97) -> (-51.5199, -97)
  arc A2 (-51.5199, -97) -> (-52.9249, -97) centre (-52.2224, -92.0496) ccw
  line L4 (-52.9249, -97) -> (-157, -97)
  arc A3 (-157, -97) -> (-154, -100) centre (-154, -97) ccw
  line L5 (-154, -100) -> (-28, -100)
  line L6 (-28, -100) -> (-25, -103)
  line L7 (-25, -103) -> (-6, -103)
  circle A4 centre (-52.2224, -92.0496) radius 3.135
  line L8 (-7, -93) -> (-7, -97) construction
  line L9 (-16, -93) -> (-16, -97) construction
  line L10 (-7, -97) -> (-16, -97)
  line L11 (-16, -97) -> (-16, -100)
  line L12 (-16, -100) -> (-7, -100)
  line L13 (-7, -100) -> (-7, -97)
  line L14 (-7, -7) -> (-7, -3) construction
  line L15 (-16, -7) -> (-16, -3) construction
  line L16 (-7, -3) -> (-16, -3)
  line L17 (-16, -3) -> (-16, 0)
  line L18 (-16, 0) -> (-7, 0)
  line L19 (-7, 0) -> (-7, -3)
  constraint coincident L3 L8.end
  constraint perpendicular L3 L8
  constraint coincident L3 L9.end
  constraint perpendicular L3 L9
  constraint horizontal L10
  constraint vertical L11
  constraint horizontal L12
  constraint vertical L13
  constraint vertical L14
  constraint vertical L15
  constraint horizontal L16
  constraint vertical L17
  constraint horizontal L18
  constraint vertical L19
extrude "Extrude23''" cut sketch "Sketch22" against normal blind 23.65 contours L3 L10 L11 L12 L13 | L16 L17 L18 L19 bodies 4 in component "Chassis"
sketch "Sketch23" plane through (3, 0, 0) normal (1, 0, 0) x (0, 0, -1) in component "Chassis"
  circle A0 centre (50, -6.65) radius 1.375
  circle A1 centre (50, -11.65) radius 1.375
  line L0 (92, -2) -> (8, -2)
  arc A2 (6, 0) -> (8, -2) centre (8, 0) ccw
  line L1 (6, 0) -> (6, -23.65)
  line L2 (6, -23.65) -> (94, -23.65)
  line L3 (94, -23.65) -> (94, 0)
  arc A3 (92, -2) -> (94, 0) centre (92, 0) ccw
  line L4 (71, -15.2) -> (61.4, -15.2)
  line L5 (61.4, -15.2) -> (61.4, -5)
  line L6 (61.4, -5) -> (71, -5)
  line L7 (71, -5) -> (71, -15.2)
  line L8 (71, -15.2) -> (61.4, -5) construction
  line L9 (61.4, -15.2) -> (71, -5) construction
  line L10 (66.2, -10.1) -> (74.85, -10.1) construction
  line L11 (66.2, -10.1) -> (57.55, -10.1) construction
  circle A4 centre (57.55, -10.1) radius 1.8
  circle A5 centre (74.85, -10.1) radius 1.8
  point P0 (66.2, -10.1)
  dimension "d437" = 9.6
  dimension "d438" = 10.2
  dimension "d439" = 3
  dimension "d440" = 23
  dimension "d441" = 8.65
  dimension "d442" = 8.65
  dimension "d443" = 3.6
  dimension "d444" = 3.6
  constraint horizontal L4
  constraint perpendicular L4 L5
  constraint parallel L4 L6
  constraint parallel L5 L7
  constraint coincident L8 P0
  constraint coincident L9 P0
  constraint coincident P0 L10.start
  constraint parallel L0 L10
  constraint perpendicular L5 L11
  constraint coincident L11.end A4.centre
  constraint coincident L10.end A5.centre
  measures "d437" distance of L5.end L6.end
  measures "d438" distance of L4.end L5.end
  measures "d439" distance of L0 L6
  measures "d440" distance of L3 L7
  measures "d441" distance of P0 L10.end
  measures "d442" distance of P0 L11.end
  measures "d443" diameter of A4
  measures "d444" diameter of A5
extrude "Extrude24'" cut sketch "Sketch23" against normal blind 3 contours L4 L5 L6 L7 | A4 | A5 bodies 4 in component "Chassis"
delete_face "DeleteFace3" 1 faces at (12.495, -29.4667, -4.0004) on bodies 15 in component "Front_R_Mounting_Plate"
delete_face "DeleteFace4" 1 faces at (12.495, -30.7833, -30.0296) on bodies 15 in component "Front_R_Mounting_Plate"
sketch "Sketch25" plane through (0, 0, 0) normal (-1, 0, 0) x (0, 0, 1) in component "Chassis"
  line L0 (-61.4, -5) -> (-61.4, -15.2)
  line L1 (-61.4, -15.2) -> (-71, -15.2)
  line L2 (-71, -15.2) -> (-71, -5)
  line L3 (-71, -5) -> (-61.4, -5)
  circle A0 centre (-57.55, -10.1) radius 1.8
  circle A1 centre (-74.85, -10.1) radius 1.8
  circle A2 centre (-50, -6.65) radius 1.375
  circle A3 centre (-50, -11.65) radius 1.375
  line L4 (-94, 0) -> (-97, 0)
  line L5 (-97, 0) -> (-97, -26.65)
  line L6 (-97, -26.65) -> (-3, -26.65)
  line L7 (-3, -26.65) -> (-3, 0)
  line L8 (-3, 0) -> (-6, 0)
  arc A4 (-8, -2) -> (-6, 0) centre (-8, 0) ccw
  line L9 (-8, -2) -> (-92, -2)
  arc A5 (-94, 0) -> (-92, -2) centre (-92, 0) ccw
  line L10 (-84.85, -2) -> (-40, -2)
  line L11 (-40, -2) -> (-40, -26.65)
  line L12 (-40, -26.65) -> (-84.85, -26.65)
  line L13 (-84.85, -26.65) -> (-84.85, -2)
  dimension "d447" = 10
  dimension "d448" = 10
  constraint horizontal L10
  constraint vertical L11
  constraint horizontal L12
  constraint vertical L13
  constraint coincident L6 L11.end
  constraint coincident L9 L10.start
  measures "d447" distance of A1.centre L13
  measures "d448" distance of A3.centre L11
extrude "Extrude25'" add sketch "Sketch25" along normal blind 5 contours L0 L1 L2 L3 | A0 | A1 | A2 | A3 | L6 L9 L10 L11 L12 L13 bodies 4 in component "Chassis"
chamfer "Chamfer5" distance 5 angle 45 2 edges at (-5, -14.325, -84.85) (-5, -14.325, -40) on bodies 4 in component "Chassis"
extrude "Extrude26" cut 5 faces at (0, -9.5804, -74.283) (0, -11.8, -64.6) (0, -10.3679, -57.1102) (0, -11.2131, -50.2352) (0, -6.2131, -50.2352) along direction (-1, 0, 0) blind 5 on bodies 4 bodies 4 in component "Chassis"
sketch "Sketch27" plane through (3, 0, 0) normal (1, 0, 0) x (0, 0, -1) in component "Chassis"
  line L0 (61.4, -15.2) -> (61.4, -5)
  line L1 (61.4, -5) -> (71, -5)
  line L2 (71, -5) -> (71, -15.2)
  line L3 (71, -15.2) -> (61.4, -15.2)
  circle A0 centre (57.55, -10.1) radius 1.8
  circle A1 centre (74.85, -10.1) radius 1.8
  circle A2 centre (50, -6.65) radius 1.375
  circle A3 centre (50, -11.65) radius 1.375
  line L4 (92, -2) -> (8, -2)
  arc A4 (6, 0) -> (8, -2) centre (8, 0) ccw
  line L5 (6, 0) -> (6, -23.65)
  line L6 (6, -23.65) -> (94, -23.65)
  line L7 (94, -23.65) -> (94, 0)
  arc A5 (92, -2) -> (94, 0) centre (92, 0) ccw
  line L8 (45, -2) -> (79.85, -2)
  line L9 (79.85, -2) -> (79.85, -23.65)
  line L10 (79.85, -23.65) -> (45, -23.65)
  line L11 (45, -23.65) -> (45, -2)
  dimension "d454" = 5
  dimension "d455" = 5
  constraint horizontal L8
  constraint vertical L9
  constraint horizontal L10
  constraint vertical L11
  constraint coincident L6 L9.end
  constraint coincident L4 L8.start
  measures "d454" distance of A1.centre L9
  measures "d455" distance of A3.centre L11
extrude "Extrude27" cut sketch "Sketch27" against normal blind 5 contours L4 L6 L8 L9 L10 L11 bodies 4 in component "Chassis"
sketch "Sketch28" plane through (0, -2, 0) normal (0, 1, 0) x (-1, 0, 0) in component "Chassis"
  line L0 (-3, -45) -> (2, -45)
  line L1 (2, -45) -> (2, -79.85)
  line L2 (2, -79.85) -> (-3, -79.85)
  line L3 (-3, -79.85) -> (-3, -92)
  line L4 (-3, -92) -> (0, -92)
  line L5 (0, -92) -> (0, -84.85)
  line L6 (0, -84.85) -> (5, -79.85)
  line L7 (5, -79.85) -> (5, -45)
  line L8 (5, -45) -> (0, -40)
  line L9 (0, -40) -> (0, -8)
  line L10 (0, -8) -> (-3, -8)
  line L11 (-3, -8) -> (-3, -45)
  line L12 (0, -84.85) -> (0, -40)
  constraint coincident L5.end L6.start
  constraint coincident L8.end L9.start
extrude "Extrude28" add sketch "Sketch28" along normal blind 1.57 contours L0 L1 L2 L6 L7 L8 L12 | L0 L1 L2 L12 bodies 4 in component "Chassis"
sketch "Sketch29" plane through (0, 0, 0) normal (0, 1, 0) x (-1, 0, 0) in component "Chassis"
  circle A0 centre (-52.2224, -92.0496) radius 3.135
  line L0 (-7, -97) -> (-7, -100)
  line L1 (-7, -100) -> (-16, -100)
  line L2 (-16, -100) -> (-16, -97)
  line L3 (-16, -97) -> (-51.5199, -97)
  arc A1 (-51.5199, -97) -> (-52.9249, -97) centre (-52.2224, -92.0496) ccw
  line L4 (-52.9249, -97) -> (-157, -97)
  arc A2 (-157, -97) -> (-154, -100) centre (-154, -97) ccw
  line L5 (-154, -100) -> (-28, -100)
  line L6 (-28, -100) -> (-25, -103)
  line L7 (-25, -103) -> (-6, -103)
  line L8 (-6, -103) -> (-3, -100)
  arc A3 (-3, -100) -> (0, -97) centre (-3, -97) ccw
  line L9 (0, -97) -> (0, -94)
  line L10 (0, -94) -> (-3, -94)
  arc A4 (-6, -97) -> (-3, -94) centre (-6, -94) ccw
  line L11 (-6, -97) -> (-7, -97)
  line L12 (-3, -100) -> (-28, -100)
  constraint coincident L8.end A3.start
  constraint coincident L5.end L6.start
extrude "Extrude29" add sketch "Sketch29" along normal blind 1.57 contours L1 L6 L7 L8 L12 bodies 4 in component "Chassis"
sketch "Sketch30" plane through (0, 0, 0) normal (0, 1, 0) x (-1, 0, 0) in component "Chassis"
  line L0 (-7, 0) -> (-7, -3)
  line L1 (-7, -3) -> (-6, -3)
  arc A0 (-3, -6) -> (-6, -3) centre (-6, -6) ccw
  line L2 (-3, -6) -> (0, -6)
  line L3 (0, -6) -> (0, -3)
  arc A1 (0, -3) -> (-3, 0) centre (-3, -3) ccw
  line L4 (-3, 0) -> (-6, 3)
  line L5 (-6, 3) -> (-25, 3)
  line L6 (-25, 3) -> (-28, 0)
  line L7 (-28, 0) -> (-154, 0)
  arc A2 (-154, 0) -> (-157, -3) centre (-154, -3) ccw
  line L8 (-157, -3) -> (-105.3473, -3)
  arc A3 (-105.3473, -3) -> (-99.7323, -3) centre (-102.5398, -7.1374) ccw
  line L9 (-99.7323, -3) -> (-16, -3)
  line L10 (-16, -3) -> (-16, 0)
  line L11 (-16, 0) -> (-7, 0)
  circle A4 centre (-102.5398, -7.1374) radius 3.135
  line L12 (-3, 0) -> (-28, 0)
  constraint coincident A1.end L4.start
  constraint coincident L6.end L7.start
extrude "Extrude30" add sketch "Sketch30" along normal blind 1.57 contours L4 L5 L6 L11 L12 bodies 4 in component "Chassis"
extrude "Extrude31" add 1 faces at (-1.6667, -0.43, -68.2333) along direction (0, 1, 0) blind 2 on bodies 4 bodies 4 in component "Chassis"
sketch "Sketch1 (10)" plane through (0, -26.65, 0) normal (0, -1, 0) x (1, 0, 0) in component "R_R_Wheel_Base"
  line L0 (0, -40) -> (-5, -45)
  line L1 (-5, -45) -> (-5, -79.85)
  line L2 (-5, -79.85) -> (0, -84.85)
  line L3 (0, -84.85) -> (0, -97)
  arc A0 (0, -97) -> (3, -100) centre (3, -97) ccw
  line L4 (3, -100) -> (6, -103)
  line L5 (6, -103) -> (25, -103)
  line L6 (25, -103) -> (28, -100)
  line L7 (28, -100) -> (154, -100)
  arc A1 (154, -100) -> (157, -97) centre (154, -97) ccw
  line L8 (157, -97) -> (157, -94)
  arc A2 (160, -91) -> (157, -94) centre (160, -94) ccw
  line L9 (160, -91) -> (181.27, -91)
  arc A3 (181.27, -91) -> (184.27, -88) centre (181.27, -88) ccw
  line L10 (184.27, -88) -> (184.27, -12)
  arc A4 (184.27, -12) -> (181.27, -9) centre (181.27, -12) ccw
  line L11 (181.27, -9) -> (160, -9)
  arc A5 (157, -6) -> (160, -9) centre (160, -6) ccw
  line L12 (157, -6) -> (157, -3)
  arc A6 (157, -3) -> (154, 0) centre (154, -3) ccw
  line L13 (154, 0) -> (28, 0)
  line L14 (28, 0) -> (25, 3)
  line L15 (25, 3) -> (6, 3)
  line L16 (6, 3) -> (3, 0)
  arc A7 (3, 0) -> (0, -3) centre (3, -3) ccw
  line L17 (0, -3) -> (0, -40)
  circle A8 centre (3, -97) radius 1.0625
  circle A9 centre (3, -71) radius 1.0625
  circle A10 centre (22, -71) radius 1.0625
  circle A11 centre (3, -29) radius 1.0625
  circle A12 centre (3, -3) radius 1.0625
  circle A13 centre (22, -29) radius 1.0625
  circle A14 centre (90, -16) radius 1.0625
  circle A15 centre (114, -16) radius 1.0625
  circle A16 centre (90, -30.28) radius 1.0625
  circle A17 centre (114, -30.28) radius 1.0625
  circle A18 centre (114, -69.72) radius 1.0625
  circle A19 centre (90, -84) radius 1.0625
  circle A20 centre (90, -69.72) radius 1.0625
  circle A21 centre (114, -84) radius 1.0625
  line L18 (92.5, -27.97) -> (92.5, -18.97)
  line L19 (92.5, -18.97) -> (112.5, -18.97)
  line L20 (112.5, -18.97) -> (112.5, -27.97)
  line L21 (112.5, -27.97) -> (92.5, -27.97)
  circle A22 centre (11.5, -70.07) radius 1
  circle A23 centre (11.5, -4.1) radius 1
  circle A24 centre (11.5, -29.93) radius 1
  line L22 (92.5, -81.36) -> (92.5, -72.36)
  line L23 (92.5, -72.36) -> (112.5, -72.36)
  line L24 (112.5, -72.36) -> (112.5, -81.36)
  line L25 (112.5, -81.36) -> (92.5, -81.36)
  circle A25 centre (89.585, -23.47) radius 1
  circle A26 centre (115.415, -76.86) radius 1
  line L26 (16, -72.97) -> (16, -93)
  line L27 (16, -93) -> (7, -93)
  line L28 (7, -93) -> (7, -72.97)
  line L29 (7, -72.97) -> (16, -72.97)
  line L30 (16, -7) -> (16, -27.03)
  line L31 (16, -27.03) -> (7, -27.03)
  line L32 (7, -27.03) -> (7, -7)
  line L33 (7, -7) -> (16, -7)
  circle A27 centre (11.5, -95.9) radius 1
  circle A28 centre (89.585, -76.86) radius 1
  circle A29 centre (115.415, -23.47) radius 1
  line L34 (127.5, -73.5) -> (124.5, -73.5)
  line L35 (124.5, -73.5) -> (124.5, -68.5)
  line L36 (124.5, -68.5) -> (127.5, -68.5)
  line L37 (127.5, -68.5) -> (127.5, -73.5)
  line L38 (183.5, -73.5) -> (180.5, -73.5)
  line L39 (180.5, -73.5) -> (180.5, -68.5)
  line L40 (180.5, -68.5) -> (183.5, -68.5)
  line L41 (183.5, -68.5) -> (183.5, -73.5)
  line L42 (127.5, -31.5) -> (124.5, -31.5)
  line L43 (124.5, -31.5) -> (124.5, -26.5)
  line L44 (124.5, -26.5) -> (127.5, -26.5)
  line L45 (127.5, -26.5) -> (127.5, -31.5)
  line L46 (183.5, -31.5) -> (180.5, -31.5)
  line L47 (180.5, -31.5) -> (180.5, -26.5)
  line L48 (180.5, -26.5) -> (183.5, -26.5)
  line L49 (183.5, -26.5) -> (183.5, -31.5)
  line L50 (36.83, -3.81) -> (36.83, -13.97)
  line L51 (36.83, -13.97) -> (19.05, -13.97)
  line L52 (19.05, -13.97) -> (19.05, -3.81)
  line L53 (19.05, -3.81) -> (36.83, -3.81)
  line L54 (36.83, -96.52) -> (19.05, -96.52)
  line L55 (19.05, -96.52) -> (19.05, -86.36)
  line L56 (19.05, -86.36) -> (36.83, -86.36)
  line L57 (36.83, -86.36) -> (36.83, -96.52)
  line L58 (114.3, -3.81) -> (130.81, -3.81)
  line L59 (130.81, -3.81) -> (130.81, -13.97)
  line L60 (130.81, -13.97) -> (114.3, -13.97)
  line L61 (114.3, -13.97) -> (114.3, -3.81)
  line L62 (114.3, -96.52) -> (114.3, -86.36)
  line L63 (114.3, -86.36) -> (130.81, -86.36)
  line L64 (130.81, -86.36) -> (130.81, -96.52)
  line L65 (130.81, -96.52) -> (114.3, -96.52)
  line L66 (89.585, -23.47) -> (115.415, -23.47) construction
  line L67 (102.5, -23.47) -> (102.5, -29.6509) construction
  line L68 (118, -16.47) -> (87, -16.47)
  line L69 (87, -16.47) -> (87, -30.47)
  line L70 (87, -30.47) -> (118, -30.47)
  line L71 (118, -30.47) -> (118, -16.47)
  line L72 (118, -16.47) -> (87, -30.47) construction
  line L73 (87, -16.47) -> (118, -30.47) construction
  point P0 (102.5, -23.47)
  dimension "d466" = 31
  dimension "d467" = 14
  constraint coincident A25.centre L66.start
  constraint coincident A29.centre L66.end
  constraint midpoint L66 P0
  constraint perpendicular L66 L67
  constraint horizontal L68
  constraint perpendicular L68 L69
  constraint parallel L68 L70
  constraint parallel L69 L71
  constraint coincident L72 P0
  constraint coincident L73 P0
  constraint coincident P0 L67.start
  measures "d466" distance of L69.end L70.end
  measures "d467" distance of L68.end L69.end